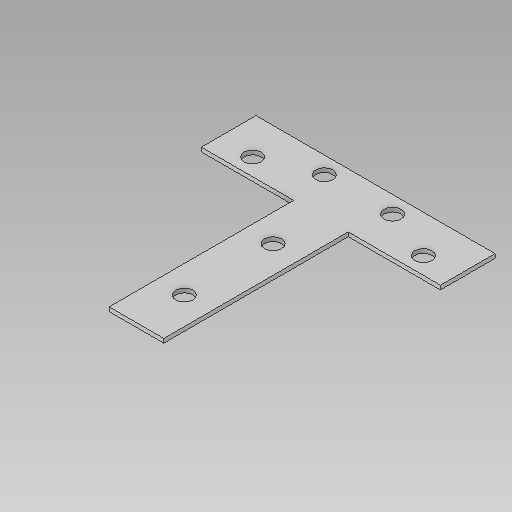
# Autodesk Inventor part: FlatTee
Saved by Autodesk Inventor 2017 (Build 210142000, 142)
## iProperties
Created: 2016-10-11
Part Number: FlatTee
Material: Generic
Document SubType Name: Modeling
Designer: krosie
Density: 1 g/cm^3
Appearance: Default
Author: krosie
Autodesk Inventor part; units mm, degrees
ref_plane "YZ Plane" through (0, 0, 0) normal (1, 0, 0) x (0, 1, 0)
ref_plane "XZ Plane" through (0, 0, 0) normal (0, 1, 0) x (-1, 0, 0)
ref_plane "XY Plane" through (0, 0, 0) normal (0, 0, 1) x (1, 0, 0)
sketch "Sketch1" plane through (0, 0, 0) normal (0, 1, 0) x (-1, 0, 0)
  line L0 (-35, 8) -> (-35, -8)
  line L1 (-35, -8) -> (35, -8)
  line L2 (35, -8) -> (35, 8)
  line L3 (35, 8) -> (-35, -8) construction
  line L4 (-35, 8) -> (35, -8) construction
  line L5 (-8, 8) -> (-8, 62)
  line L6 (-8, 62) -> (8, 62)
  line L7 (8, 62) -> (8, 8)
  line L8 (0, 0) -> (0, 99.8973) construction
  line L9 (35, 8) -> (8, 8)
  line L10 (-8, 8) -> (-35, 8)
  circle A0 centre (25, 3) radius 2.5
  circle A1 centre (10, -3) radius 2.5
  circle A2 centre (-10, -3) radius 2.5
  circle A3 centre (-25, 3) radius 2.5
  circle A4 centre (0, 22) radius 2.5
  circle A5 centre (0, 48) radius 2.5
  dimension "d0" = 70
  dimension "d1" = 16
  dimension "d2" = 16
  dimension "d4" = 70
  dimension "d5" = 5
  dimension "d6" = 5
  dimension "d7" = 5
  dimension "d8" = 10
  dimension "d10" = 10
  dimension "d11" = 10
  dimension "d12" = 10
  dimension "d13" = 14
  dimension "d14" = 40
  constraints: 22 end point, 6 centre point, 5 equal radius, 4 parallel, 2 horizontal, 2 horizontal alignment, 2 midpoint, 2 perpendicular, 1 collinear, 1 point on line, 1 vertical, 1 vertical alignment, 1 other
  measures "d0" distance of L1.end L0.end
  measures "d1" distance of L0.end L0.start
  measures "d2" distance of L5.end L6.end
  measures "d4" distance between parallel lines of L1 L6
  measures "d5" diameter of A3
  measures "d6" distance from line of L10 A3.centre
  measures "d7" distance from line of L1 A2.centre
  measures "d8" distance from line of L2 A0.centre
  measures "d10" distance from line of L8 A1.centre
  measures "d11" distance from line of A2.centre L8
  measures "d12" distance from line of L0 A3.centre
  measures "d13" distance from line of L6 A5.centre
  measures "d14" distance from line of L6 A4.centre
extrude "Extrusion1" add sketch "Sketch1" along normal blind 1.2
equation "\"d10\" = d8"
equation "\"d11\" = d8"
equation "\"d12\" = d8"
equation "\"d13\" = 0.2 * d4"
equation "\"d14\" = 0.571429 * d4"
body "Solid1"
